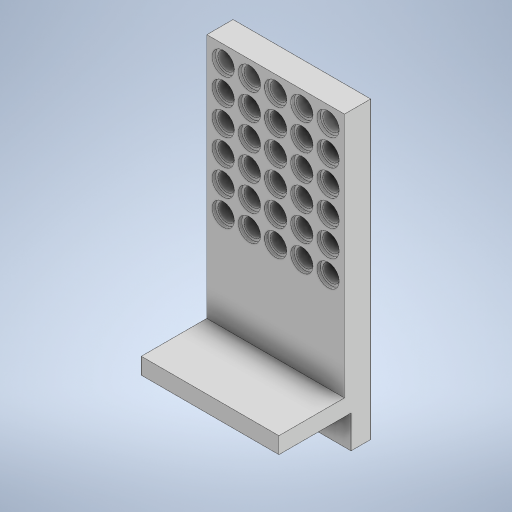
# Autodesk Inventor part: derocana_deska
Saved by Autodesk Inventor 2024.2 (Build 282272000, 272)
## iProperties
Created: 2024-01-18
Part Number: derocana_deska
Material: Generic
Document SubType Name: Modeling
Designer: filip
Density: 1 g/cm^3
Appearance: Default
Author: filip
Autodesk Inventor part; units mm, degrees
ref_plane "YZ Plane" through (0, 0, 0) normal (1, 0, 0) x (0, 1, 0)
ref_plane "XZ Plane" through (0, 0, 0) normal (0, 1, 0) x (-1, 0, 0)
ref_plane "XY Plane" through (0, 0, 0) normal (0, 0, 1) x (1, 0, 0)
sketch "Sketch1" plane through (0, 0, 0) normal (0, 0, 1) x (1, 0, 0)
  line L0 (21, -40) -> (-21, -40)
  line L1 (-21, -40) -> (-21, 40)
  line L2 (-21, 40) -> (21, 40)
  line L3 (21, 40) -> (21, -40)
  line L4 (21, -40) -> (-21, 40) construction
  line L5 (-21, -40) -> (21, 40) construction
  point P0 (0, 0)
  dimension "d0" = 42
  dimension "d1" = 80
  constraints: 12 end point, 2 midpoint, 2 parallel, 1 horizontal, 1 perpendicular
  measures "d0" distance of L1.end L2.end
  measures "d1" distance of L0.end L1.end
extrude "Extrusion1" add sketch "Sketch1" along normal blind 8
sketch "Sketch2" plane through (0, 0, 8) normal (0, 0, 1) x (1, 0, 0)
  line L0 (-21, 40) -> (-21, -40) projected
  line L1 (21, 40) -> (-21, 40) projected
  point P0 (0, 0)
  point P1 (-16, 35)
  dimension "d4" = 5
  dimension "d5" = 5
  measures "d4" distance from line of L0 point (-16, 35)
  measures "d5" distance from line of L1 point (-16, 35)
hole "Hole1" at (-16, 35, 8) direction (0, 0, -1) diameter 5.3 end through all counterbore diameter 6.8 counterbore depth 1
pattern_linear "Rectangular Pattern1" count 6 spacing 8 along (0, -1, 0) count 5 spacing 8 along (1, 0, 0) of "Hole1"
sketch "Sketch3" plane through (0, 0, 8) normal (0, 0, 1) x (1, 0, 0)
  line L0 (-21, 40) -> (-21, -40) projected
  line L1 (21, -40) -> (21, 40) projected
  line L2 (-21, -40) -> (21, -40)
  line L3 (21, -40) -> (21, -35)
  line L4 (21, -35) -> (-21, -35)
  line L5 (-21, -35) -> (-21, -40)
  point P0 (0, 0)
  dimension "d19" = 5
  constraints: 8 end point, 2 parallel, 1 horizontal, 1 perpendicular, 1 point on line
  measures "d19" distance of L3.end L2.end
extrude "Extrusion2" add sketch "Sketch3" along normal blind 20
sketch "Sketch4" plane through (-21, -40, 0) normal (0, -1, 0) x (1, 0, 0)
  line L0 (0, 0) -> (0, 8) projected
  line L1 (42, 0) -> (42, 8) projected
  line L2 (0, 0) -> (42, 0)
  line L3 (42, 0) -> (42, 6)
  line L4 (42, 6) -> (0, 6)
  line L5 (0, 6) -> (0, 0)
  point P0 (21, 0)
  point P1 (0, 6)
  dimension "d22" = 6
  constraints: 8 end point, 2 parallel, 1 horizontal, 1 perpendicular, 1 point on line
  measures "d22" distance of L3.end L2.end
extrude "Extrusion3" add sketch "Sketch4" along normal blind 10
fillet "Fillet1" [suppressed]
sketch "Sketch5" plane through (0, 0, 0) normal (0, 0, -1) x (-1, 0, 0)
  circle A0 centre (16, 35) radius 3.4 projected
  point P0 (0, 0)
extrude "Extrusion4" cut sketch "Sketch5" against normal blind 1
pattern_linear "Rectangular Pattern2" count 5 spacing 8 along (1, 0, 0) count 6 spacing 8 along (0, -1, 0) of "Extrusion4"
body "Solid1"
